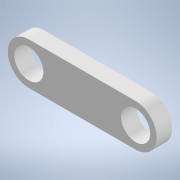
# Autodesk Inventor part: IntakeChainLink
Saved by Autodesk Inventor 2020 (Build 240168000, 168)
## iProperties
Created: 2020-01-19
Part Number: IntakeChainLink
Material: Generic
Document SubType Name: Modeling
Designer: srini
Density: 1 g/cm^3
Appearance: Default
Author: srini
Autodesk Inventor part; units mm, degrees
ref_plane "YZ Plane" through (0, 0, 0) normal (1, 0, 0) x (0, 1, 0)
ref_plane "XZ Plane" through (0, 0, 0) normal (0, 1, 0) x (-1, 0, 0)
ref_plane "XY Plane" through (0, 0, 0) normal (0, 0, 1) x (1, 0, 0)
sketch "Sketch1" plane through (0, 0, 0) normal (0, 0, 1) x (1, 0, 0)
  line L0 (-52.3875, 0) -> (52.3875, 0) construction
  line L1 (-52.3875, -20.6502) -> (52.3875, -20.6502)
  line L2 (52.3875, 20.6502) -> (-52.3875, 20.6502)
  arc A0 (-52.3875, 20.6502) -> (-52.3875, -20.6502) centre (-52.3875, 0) ccw
  arc A1 (52.3875, -20.6502) -> (52.3875, 20.6502) centre (52.3875, 0) ccw
  point P0 (0, 0)
  dimension "d0" = 104.775
  dimension "d1" = 20.6502
  constraints: 8 end point, 4 point on circle, 4 tangent, 2 centre point, 1 horizontal, 1 midpoint, 1 parallel
  measures "d0" distance of L0.start L0.end
  measures "d1" radius of A0
extrude "Extrusion1" add sketch "Sketch1" along normal blind 15.24
sketch "Sketch2" plane through (0, 0, 15.24) normal (0, 0, 1) x (1, 0, 0)
  arc A0 (-52.3875, 20.6502) -> (-52.3875, -20.6502) centre (-52.3875, 0) ccw projected
  circle A1 centre (-52.3875, 0) radius 14.3002
  arc A2 (52.3875, -20.6502) -> (52.3875, 20.6502) centre (52.3875, 0) ccw projected
  circle A3 centre (52.3875, 0) radius 14.3002
  point P0 (0, 0)
  dimension "d4" = 28.6004
  constraints: 2 centre point, 2 coincident, 1 equal radius
  measures "d4" diameter of A1
extrude "Extrusion2" cut sketch "Sketch2" against normal through all
body "Solid1"
